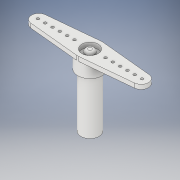
# Autodesk Inventor part: Servo shaft and horn
Saved by Autodesk Inventor 2018 (Build 220112000, 112)
## iProperties
Created: 2018-06-25
Part Number: Servo shaft and horn
Material: Generic
Document SubType Name: Modeling
Designer: Ajith Thomas
Density: 1 g/cm^3
Appearance: White
Author: Ajith Thomas
Autodesk Inventor part; units mm, degrees
ref_plane "YZ Plane" through (0, 0, 0) normal (1, 0, 0) x (0, 1, 0)
ref_plane "XZ Plane" through (0, 0, 0) normal (0, 1, 0) x (-1, 0, 0)
ref_plane "XY Plane" through (0, 0, 0) normal (0, 0, 1) x (1, 0, 0)
sketch "Sketch1" plane through (0, 0, 0) normal (0, 1, 0) x (-1, 0, 0)
  circle A0 centre (0, 0) radius 2.5
  dimension "d0" = 5
  constraints: 1 centre point, 1 coincident
  measures "d0" diameter of A0
extrude "Extrusion1" add sketch "Sketch1" along normal blind 9.5 and the other way blind 10
sketch "Sketch2" plane through (0, 9.5, 0) normal (0, 1, 0) x (1, 0, 0)
  line L0 (0, 0) -> (-16, 0) construction
  line L1 (0, 0) -> (0, 3.35) construction
  arc A0 (-14.1929, 1.9907) -> (-14.1929, -1.9907) centre (-14, 0) ccw
  line L2 (-14.1929, -1.9907) -> (-0.323, -3.3344)
  line L3 (-14.1929, 1.9907) -> (-0.323, 3.3344)
  arc A1 (14.1929, -1.9907) -> (14.1929, 1.9907) centre (14, 0) ccw
  line L4 (14.1929, -1.9907) -> (0.323, -3.3344)
  line L5 (14.1929, 1.9907) -> (0.323, 3.3344)
  circle A2 centre (0, 0) radius 2.5
  arc A3 (-0.323, -3.3344) -> (0.323, -3.3344) centre (0, 0) ccw
  arc A4 (0.323, 3.3344) -> (-0.323, 3.3344) centre (0, 0) ccw
  dimension "d5" = 16
  dimension "d7" = 4
  dimension "d8" = 2
  dimension "d11" = 0.85
  constraints: 12 end point, 9 point on circle, 5 centre point, 5 symmetric about line, 4 tangent, 2 coincident, 1 horizontal, 1 point on line, 1 vertical, 1 other
  measures "d5" distance of L0.start L0.end
  measures "d7" diameter of A0
  measures "d8" distance of A0.centre L0.end
  measures "d11" radial gap between concentric circles of A2 A4
extrude "Extrusion2" add sketch "Sketch2" against normal blind 1.2
sketch "Sketch3" plane through (0, 8.3, 0) normal (0, -1, 0) x (1, 0, 0)
  circle A0 centre (0, 0) radius 2.5 projected
  circle A1 centre (0, 0) radius 3.35
  constraints: 1 centre point, 1 coincident
extrude "Extrusion3" add sketch "Sketch3" along normal blind 3.5
sketch "Sketch4" plane through (0, 9.5, 0) normal (0, 1, 0) x (1, 0, 0)
  circle A0 centre (0, 0) radius 2.25
  dimension "d16" = 4.5
  constraints: 1 centre point, 1 coincident
  measures "d16" diameter of A0
extrude "Extrusion4" cut sketch "Sketch4" against normal blind 1.25
sketch "Sketch5" plane through (0, 8.25, 0) normal (0, 1, 0) x (1, 0, 0)
  circle A0 centre (0, 0) radius 1.25
  dimension "d19" = 2.5
  constraints: 1 centre point, 1 coincident
  measures "d19" diameter of A0
extrude "Extrusion5" add sketch "Sketch5" along normal blind 1.25
fillet "Fillet1" radius 0.74 1 edges at (-1.25, 9.5, 0)
sketch "Sketch6" plane through (0, 9.5, 0) normal (0, 1, 0) x (1, 0, 0)
  circle A0 centre (-4.25, 0) radius 0.375
  line L0 (0, 0) -> (-16, 0) construction
  arc A1 (-14.1929, 1.9907) -> (-14.1929, -1.9907) centre (-14, 0) ccw construction
  circle A2 centre (-6.25, 0) radius 0.375
  circle A3 centre (-8.25, 0) radius 0.375
  circle A4 centre (-10.25, 0) radius 0.375
  circle A5 centre (-12.25, 0) radius 0.375
  circle A6 centre (-14.25, 0) radius 0.375
  dimension "d23" = 0.75
  dimension "d24" = 4.25
  dimension "d27" = 2
  constraints: 6 centre point, 2 end point, 2 horizontal, 1 point on circle, 10 other
  measures "d23" diameter of A0
  measures "d24" distance of L0.start A0.centre
  measures "d27" distance of A0.centre A2.centre
extrude "Extrusion6" cut sketch "Sketch6" against normal blind 2.8375
mirror "Mirror1" about plane through (0, 0, 0) normal (1, 0, 0) of "Extrusion6"
body "Solid1"
